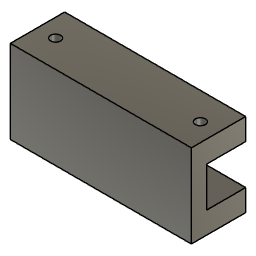
table-attachment (Autodesk Fusion 360 design; units mm, degrees)
Autodesk Fusion 360 part; units mm, degrees
sketch "main" plane through (0, 0, 0) normal (0, 0, 1) x (1, 0, 0)
  line L0 (-50, 15) -> (50, 15)
  line L1 (50, 15) -> (50, -15)
  line L2 (50, -15) -> (-50, -15)
  line L3 (-50, -15) -> (-50, 15)
  line L4 (-50, 15) -> (50, -15) construction
  line L5 (50, 15) -> (-50, -15) construction
  line L6 (30, 15) -> (-30, 15) construction
  line L7 (-30, 15) -> (-30, -15) construction
  line L8 (-30, -15) -> (30, -15) construction
  line L9 (30, -15) -> (30, 15) construction
  line L10 (-50, 15) -> (-30, -15) construction
  line L11 (-30, 15) -> (-50, -15) construction
  circle A0 centre (-40, 0) radius 2.75
  line L12 (30, 15) -> (50, -15) construction
  line L13 (50, 15) -> (30, -15) construction
  circle A1 centre (40, 0) radius 2.75
  line L14 (-50, -15) -> (50, -15)
  line L15 (50, -15) -> (50, -6.5)
  line L16 (50, -6.5) -> (-50, -6.5)
  line L17 (-50, -6.5) -> (-50, -15)
  line L18 (35.95, -4.05) -> (44.05, -4.05)
  line L19 (44.05, -4.05) -> (44.05, 4.05)
  line L20 (44.05, 4.05) -> (35.95, 4.05)
  line L21 (35.95, 4.05) -> (35.95, -4.05)
  line L22 (35.95, -4.05) -> (44.05, 4.05) construction
  line L23 (44.05, -4.05) -> (35.95, 4.05) construction
  line L24 (-44.05, -4.05) -> (-35.95, -4.05)
  line L25 (-35.95, -4.05) -> (-35.95, 4.05)
  line L26 (-35.95, 4.05) -> (-44.05, 4.05)
  line L27 (-44.05, 4.05) -> (-44.05, -4.05)
  line L28 (-44.05, -4.05) -> (-35.95, 4.05) construction
  line L29 (-35.95, -4.05) -> (-44.05, 4.05) construction
  line L30 (44.05, 4.05) -> (35.95, 4.05)
  line L31 (35.95, 4.05) -> (35.95, 15)
  line L32 (35.95, 15) -> (44.05, 15)
  line L33 (44.05, 15) -> (44.05, 4.05)
  line L34 (-35.95, 4.05) -> (-44.05, 4.05)
  line L35 (-44.05, 4.05) -> (-44.05, 15)
  line L36 (-44.05, 15) -> (-35.95, 15)
  line L37 (-35.95, 15) -> (-35.95, 4.05)
  point P0 (40, 0)
  point P1 (-40, 0)
  dimension "d1" = 100
  dimension "d2" = 30
  dimension "d3" = 60
  dimension "d4" = 30
  dimension "d5" = 5.5
  dimension "d6" = 5.5
  dimension "d7" = 100
  dimension "d8" = 8.5
  dimension "d17" = 8.1
  dimension "d18" = 8.1
  dimension "d19" = 8.1
  dimension "d20" = 8.1
  dimension "d21" = 8.1
  dimension "d22" = 10.95
  dimension "d23" = 8.1
  dimension "d24" = 10.95
  constraint horizontal L0
  constraint perpendicular L0 L1
  constraint parallel L0 L2
  constraint parallel L1 L3
  constraint coincident L4 origin
  constraint coincident L5 origin
  constraint horizontal L6
  constraint perpendicular L6 L7
  constraint parallel L6 L8
  constraint parallel L7 L9
  constraint midpoint L11 P1
  constraint midpoint L12 P0
  constraint horizontal L14
  constraint vertical L15
  constraint horizontal L16
  constraint vertical L17
  constraint horizontal L18
  constraint perpendicular L18 L19
  constraint parallel L18 L20
  constraint parallel L19 L21
  constraint coincident L22 P0
  constraint coincident L23 P0
  constraint coincident P0 A1.centre
  constraint horizontal L24
  constraint perpendicular L24 L25
  constraint parallel L24 L26
  constraint parallel L25 L27
  constraint coincident L28 P1
  constraint coincident L29 P1
  constraint coincident P1 A0.centre
  constraint horizontal L30
  constraint vertical L31
  constraint horizontal L32
  constraint vertical L33
  constraint horizontal L34
  constraint vertical L35
  constraint horizontal L36
  constraint vertical L37
  measures "d1" distance of L1.end L2.end
  measures "d2" distance of L0.end L1.end
  measures "d3" distance of L7.end L8.end
  measures "d4" distance of L6.end L7.end
  measures "d5" diameter of A0
  measures "d6" diameter of A1
  measures "d7" distance of L2.end L1.end
  measures "d8" distance of L2.end L16.end
  measures "d17" distance of L19.end L20.end
  measures "d18" distance of L18.end L19.end
  measures "d19" distance of L25.end L26.end
  measures "d20" distance of L24.end L25.end
  measures "d21" distance of L19.end L20.end
  measures "d22" distance of L19.end L32.end
  measures "d23" distance of L25.end L26.end
  measures "d24" distance of L25.end L36.end
extrude "Extrude1" add sketch "main" against normal blind 12
extrude "Extrude2" add sketch "main" against normal blind 22 from surface at -12 contours L1 L2 L3 L14 L15 L16 L17
extrude "Extrude3" add sketch "main" against normal blind 12 from surface at -34 contours L0 L1 L3 L16 L18 L19 L21 L24 L25 L27 L31 L33 L35 L37 | L0 L26 L34 L35 L36 L37 | L1 L2 L3 L14 L15 L16 L17 | L24 L25 L26 L27 L34 | L0 L20 L30 L31 L32 L33 | L18 L19 L20 L21 L30 | A0 | A1
extrude "Extrude4" cut sketch "main" along normal mid plane 3.7 from surface at -6 contours L0 L26 L34 L35 L36 L37 | L24 L25 L26 L27 L34 | L0 L20 L30 L31 L32 L33 | L18 L19 L20 L21 L30
equation "d5 = ( 2.75 * 2 ) * 1 mm"
equation "d14 = -22 mm - 12 mm"
